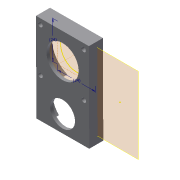
# Autodesk Inventor part: 200_Gearbox_conterplate
Saved by Autodesk Inventor 2019 (Build 230136000, 136)
## iProperties
Created: 2019-07-08
Part Number: 200_Gearbox_conterplate
Material: Generic
Document SubType Name: Modeling
Designer: diederichbenedict
Density: 1 g/cm^3
Appearance: Default
Author: diederichbenedict
Autodesk Inventor part; units mm, degrees
ref_plane "YZ Plane" through (0, 0, 0) normal (1, 0, 0) x (0, 1, 0)
ref_plane "XZ Plane" through (0, 0, 0) normal (0, 1, 0) x (-1, 0, 0)
ref_plane "XY Plane" through (0, 0, 0) normal (0, 0, 1) x (1, 0, 0)
ref_plane "Work Plane1" through (0, 0, 0) normal (0, 0, 1) x (1, 0, 0)
ref_plane "Work Plane2" through (-27.9392, 13.2515, 3.3744) normal (0, 0, 1) x (0.9999936, 0.0035868, 0)
sketch "Sketch4" plane through (-27.9392, 13.2515, 3.3744) normal (0, 0, 1) x (0.9999936, 0.0035868, 0)
  circle A0 centre (0.0013, -0.0001) radius 12.5 construction
  line L0 (15.0013, 14.9999) -> (-14.9987, 14.9999) construction
  line L1 (-14.9987, 14.9999) -> (-14.9987, -40.0001) construction
  line L2 (-14.9987, -40.0001) -> (15.0013, -40.0001) construction
  line L3 (15.0013, -40.0001) -> (15.0013, 14.9999) construction
  line L4 (15.0013, 14.9999) -> (-14.9987, 14.9999)
  line L5 (-14.9987, 14.9999) -> (-14.9987, -40.0001)
  line L6 (-14.9987, -40.0001) -> (15.0013, -40.0001)
  line L7 (15.0013, -40.0001) -> (15.0013, 14.9999)
  circle A1 centre (0.0013, -0.0001) radius 10.3271
  circle A2 centre (-0.1451, -29.1987) radius 12.8 construction
  circle A3 centre (-0.1034, -29.1986) radius 8.1726 construction
  circle A4 centre (-0.1034, -29.1986) radius 8
  point P0 (27.8915, -13.3516)
  dimension "d13" = 15
  dimension "d14" = 15
  dimension "d15" = 15
  dimension "d16" = 40
  dimension "d17" = 16
  constraints: 16 end point, 4 parallel, 3 centre point, 2 coincident, 2 horizontal, 2 perpendicular
  measures "d13" distance from line of A0.centre L3
  measures "d14" distance from line of L1 A0.centre
  measures "d15" distance from line of A0.centre L0
  measures "d16" distance from line of A0.centre L2
  measures "d17" diameter of A4
extrude "Extrusion4" add sketch "Sketch4" along normal blind 2
sketch "Sketch5" plane through (-27.9392, 13.2515, 3.3744) normal (0, 0, -1) x (-0.9999936, -0.0035868, 0)
  line L0 (15.2891, -0.4637) -> (15.1772, -1.9039) construction
  circle A0 centre (-0.0013, -0.0001) radius 12.5 construction
  line L1 (15.4007, -29.1278) -> (15.3392, -30.5711) construction
  circle A1 centre (-0.0013, -0.0001) radius 10.3271 construction
  circle A2 centre (0.1034, -29.1986) radius 8 construction
  line L2 (-15.0013, 14.9999) -> (14.9987, 14.9999) construction
  line L3 (-15.0013, -40.0001) -> (-15.0013, 14.9999) construction
  line L4 (14.9987, -40.0001) -> (-15.0013, -40.0001) construction
  line L5 (14.9987, 14.9999) -> (14.9987, -40.0001) construction
  line L6 (-15.0013, -40.0001) -> (14.9987, -40.0001)
  circle A3 centre (-0.0013, -0.0001) radius 15.2975 construction
  line L7 (14.9987, -40.0001) -> (-15.0013, -40.0001) projected
  line L8 (14.9987, 14.9999) -> (14.9987, -40.0001) projected
  line L9 (-15.0013, -40.0001) -> (-15.0013, 14.9999) projected
  line L10 (14.9987, 4.9557) -> (14.9987, 14.9999)
  arc A4 (5.9476, -14.6347) -> (14.9987, -4.956) centre (-0.0013, -0.0001) ccw
  line L11 (14.9987, -40.0001) -> (14.9987, -34.1376)
  line L12 (14.9987, -24.2596) -> (14.9987, -4.956)
  arc A5 (14.9987, -24.2596) -> (5.9476, -14.6347) centre (0.1034, -29.1986) ccw
  arc A6 (11.4871, -40.0001) -> (14.9987, -34.1376) centre (0.1034, -29.1986) ccw
  line L13 (-15.0013, 4.9557) -> (-15.0013, -4.956)
  line L14 (-15.0013, -33.4542) -> (-15.0013, -40.0001)
  arc A7 (-5.1414, -14.4082) -> (-15.0013, -24.943) centre (0.1034, -29.1986) ccw
  arc A8 (-15.0013, -33.4542) -> (-11.2803, -40.0001) centre (0.1034, -29.1986) ccw
  arc A9 (-15.0013, -4.956) -> (-5.8452, -14.677) centre (-0.0013, -0.0001) ccw
  arc A10 (14.9987, 4.9557) -> (4.9545, 14.9999) centre (-0.0013, -0.0001) ccw
  arc A11 (-4.9572, 14.9999) -> (-15.0013, 4.9557) centre (-0.0013, -0.0001) ccw
  line L15 (14.9987, 14.9999) -> (3.0009, 14.9999)
  line L16 (-3.0035, 14.9999) -> (-15.0013, 14.9999)
  line L17 (-15.0013, -4.956) -> (-15.0013, -24.943)
  line L18 (14.9987, -4.956) -> (14.9987, -24.2596)
  point P0 (-27.8915, -13.3516)
  point P1 (10.9564, -8.3909)
  constraints: 21 point on circle, 20 end point, 11 point on line, 9 centre point, 8 parallel, 4 perpendicular, 2 coincident, 2 collinear, 2 horizontal, 1 other
extrude "Extrusion5" add sketch "Sketch5" along normal blind 7
sketch "Sketch6" plane through (-27.9392, 13.2515, -3.6256) normal (0, 0, -1) x (-0.9999936, -0.0035868, 0)
  line L0 (-15.0013, -40.0001) -> (-11.2803, -40.0001) projected
  arc A0 (-5.8452, -14.677) -> (-15.0013, -24.943) centre (0.1034, -29.1986) ccw projected
  line L1 (-15.0013, -33.4542) -> (-15.0013, -40.0001) projected
  line L2 (-15.0013, -4.956) -> (-15.0013, -24.943) projected
  line L3 (14.9987, -40.0001) -> (14.9987, -34.1376) projected
  line L4 (11.4871, -40.0001) -> (14.9987, -40.0001) projected
  arc A1 (-15.0013, -33.4542) -> (-11.2803, -40.0001) centre (0.1034, -29.1986) ccw projected
  arc A2 (-4.9572, 14.9999) -> (-15.0013, 4.9557) centre (-0.0013, -0.0001) ccw projected
  line L5 (-4.9572, 14.9999) -> (-15.0013, 14.9999) projected
  line L6 (-15.0013, 14.9999) -> (-15.0013, 4.9557) projected
  arc A3 (11.4871, -40.0001) -> (14.9987, -34.1376) centre (0.1034, -29.1986) ccw projected
  arc A4 (-15.0013, -4.956) -> (-5.8452, -14.677) centre (-0.0013, -0.0001) ccw projected
  line L7 (-12.0013, 11.9999) -> (11.9987, 11.9999) construction
  line L8 (11.9987, 11.9999) -> (11.9987, -12.0001) construction
  line L9 (11.9987, -12.0001) -> (-12.0013, -12.0001) construction
  line L10 (-12.0013, -12.0001) -> (-12.0013, 11.9999) construction
  line L11 (-12.0013, 11.9999) -> (11.9987, -12.0001) construction
  line L12 (11.9987, 11.9999) -> (-12.0013, -12.0001) construction
  dimension "d32" = 24
  dimension "d33" = 24
  constraints: 12 end point, 2 midpoint, 2 parallel, 1 horizontal, 1 perpendicular
  measures "d32" distance of L8.end L9.end
  measures "d33" distance of L7.end L8.end
hole "Hole1" at (-39.9809, 25.2083, -3.6256) at (-39.8948, 1.2084, -3.6256) at (-15.895, 1.2945, -3.6256) at (-15.981, 25.2943, -3.6256) direction (0, 0, 1) diameter 2 depth 24 tip angle 118
sketch "Sketch7" plane through (-27.9392, 13.2515, -3.6256) normal (0, 0, -1) x (-0.9999936, -0.0035868, 0)
  circle A0 centre (-0.0013, -0.0001) radius 10.3271 projected
  line L0 (-12.0013, 11.9999) -> (11.9987, 11.9999) construction
  line L1 (11.9987, 11.9999) -> (11.9987, -12.0001) construction
  line L2 (11.9987, -12.0001) -> (-12.0013, -12.0001) construction
  line L3 (-12.0013, -12.0001) -> (-12.0013, 11.9999) construction
  line L4 (-12.0013, 11.9999) -> (11.9987, -12.0001) construction
  line L5 (11.9987, 11.9999) -> (-12.0013, -12.0001) construction
  point P0 (-27.8915, -13.3516)
  dimension "d30" = 24
  dimension "d31" = 24
  constraints: 12 end point, 2 midpoint, 2 parallel, 1 horizontal, 1 perpendicular
  measures "d30" distance of L1.end L2.end
  measures "d31" distance of L0.end L1.end
body "Solid2"
